Autodesk Inventor part; units mm, degrees
(part 3 of 4)
  line L1059 (-6.67, 65.7894) -> (-6.9506, 66.0778) construction
  line L1060 (-6.9506, 66.0778) -> (-7.1688, 66.0778) construction
  spline S276 degree 2 poles (-8.1665, 63.3342) (-8.1665, 63.2173) (-8.2366, 63.1472) knots 0 0 0 1 1 1
  line L1061 (-8.1665, 63.3342) -> (-8.1665, 63.2173) construction
  line L1062 (-8.1665, 63.2173) -> (-8.2366, 63.1472) construction
  spline S277 degree 2 poles (-8.2366, 63.1472) (-8.3068, 63.0848) (-8.4159, 63.0848) knots 0 0 0 1 1 1
  line L1063 (-8.2366, 63.1472) -> (-8.3068, 63.0848) construction
  line L1064 (-8.3068, 63.0848) -> (-8.4159, 63.0848) construction
  spline S278 degree 2 poles (-8.4159, 63.0848) (-8.5172, 63.0848) (-8.6653, 63.2095) (-8.6653, 63.3342) knots 0 0 0 1 2 2 2
  line L1065 (-8.4159, 63.0848) -> (-8.5172, 63.0848) construction
  line L1066 (-8.5172, 63.0848) -> (-8.6653, 63.2095) construction
  line L1067 (-8.6653, 63.2095) -> (-8.6653, 63.3342) construction
  line L1068 (-8.6653, 63.3342) -> (-8.6653, 66.3272)
  spline S279 degree 2 poles (-8.6653, 66.3272) (-8.6653, 66.5766) (-8.4159, 66.5766) knots 0 0 0 1 1 1
  line L1069 (-8.6653, 66.3272) -> (-8.6653, 66.5766) construction
  line L1070 (-8.6653, 66.5766) -> (-8.4159, 66.5766) construction
  line L1071 (-8.4159, 66.5766) -> (-7.1688, 66.5766)
  spline S280 degree 2 poles (-7.1688, 66.5766) (-6.7713, 66.5766) (-6.1712, 66.0038) (-6.1712, 65.579) knots 0 0 0 1 2 2 2
  line L1072 (-7.1688, 66.5766) -> (-6.7713, 66.5766) construction
  line L1073 (-6.7713, 66.5766) -> (-6.1712, 66.0038) construction
  line L1074 (-6.1712, 66.0038) -> (-6.1712, 65.579) construction
  line L1075 (-6.1712, 65.579) -> (-6.1712, 63.3342)
  spline S281 degree 2 poles (-6.1712, 63.3342) (-6.1712, 63.2173) (-6.2413, 63.1472) knots 0 0 0 1 1 1
  line L1076 (-6.1712, 63.3342) -> (-6.1712, 63.2173) construction
  line L1077 (-6.1712, 63.2173) -> (-6.2413, 63.1472) construction
  spline S282 degree 2 poles (2.309, 64.0825) (2.309, 63.872) (2.4532, 63.7278) knots 0 0 0 1 1 1
  line L1078 (2.309, 64.0825) -> (2.309, 63.872) construction
  line L1079 (2.309, 63.872) -> (2.4532, 63.7278) construction
  spline S283 degree 2 poles (2.4532, 63.7278) (2.5272, 63.6616) (2.6129, 63.6187) knots 0 0 0 1 1 1
  line L1080 (2.4532, 63.7278) -> (2.5272, 63.6616) construction
  line L1081 (2.5272, 63.6616) -> (2.6129, 63.6187) construction
  spline S284 degree 2 poles (2.6129, 63.6187) (2.7182, 63.5836) (2.8078, 63.5836) knots 0 0 0 1 1 1
  line L1082 (2.6129, 63.6187) -> (2.7182, 63.5836) construction
  line L1083 (2.7182, 63.5836) -> (2.8078, 63.5836) construction
  line L1084 (2.8078, 63.5836) -> (4.0549, 63.5836)
  spline S285 degree 2 poles (4.0549, 63.5836) (4.1601, 63.5836) (4.3043, 63.4317) (4.3043, 63.3342) knots 0 0 0 1 2 2 2
  line L1085 (4.0549, 63.5836) -> (4.1601, 63.5836) construction
  line L1086 (4.1601, 63.5836) -> (4.3043, 63.4317) construction
  line L1087 (4.3043, 63.4317) -> (4.3043, 63.3342) construction
  spline S286 degree 2 poles (4.3043, 63.3342) (4.3043, 63.2485) (4.1796, 63.0848) (4.0549, 63.0848) knots 0 0 0 1 2 2 2
  line L1088 (4.3043, 63.3342) -> (4.3043, 63.2485) construction
  line L1089 (4.3043, 63.2485) -> (4.1796, 63.0848) construction
  line L1090 (4.1796, 63.0848) -> (4.0549, 63.0848) construction
  line L1091 (4.0549, 63.0848) -> (2.8078, 63.0848)
  spline S287 degree 2 poles (2.8078, 63.0848) (2.4025, 63.0848) (1.8101, 63.6655) (1.8101, 64.0825) knots 0 0 0 1 2 2 2
  line L1092 (2.8078, 63.0848) -> (2.4025, 63.0848) construction
  line L1093 (2.4025, 63.0848) -> (1.8101, 63.6655) construction
  line L1094 (1.8101, 63.6655) -> (1.8101, 64.0825) construction
  line L1095 (1.8101, 64.0825) -> (1.8101, 65.579)
  spline S288 degree 2 poles (1.8101, 65.579) (1.8101, 65.9804) (2.3869, 66.5766) (2.8078, 66.5766) knots 0 0 0 1 2 2 2
  line L1096 (1.8101, 65.579) -> (1.8101, 65.9804) construction
  line L1097 (1.8101, 65.9804) -> (2.3869, 66.5766) construction
  line L1098 (2.3869, 66.5766) -> (2.8078, 66.5766) construction
  line L1099 (2.8078, 66.5766) -> (3.3066, 66.5766)
  spline S289 degree 2 poles (3.3066, 66.5766) (3.7119, 66.5766) (4.3043, 65.996) (4.3043, 65.579) knots 0 0 0 1 2 2 2
  line L1100 (3.3066, 66.5766) -> (3.7119, 66.5766) construction
  line L1101 (3.7119, 66.5766) -> (4.3043, 65.996) construction
  line L1102 (4.3043, 65.996) -> (4.3043, 65.579) construction
  line L1103 (4.3043, 65.579) -> (4.3043, 64.8307)
  spline S290 degree 2 poles (4.3043, 64.8307) (4.3043, 64.5813) (4.0549, 64.5813) knots 0 0 0 1 1 1
  line L1104 (4.3043, 64.8307) -> (4.3043, 64.5813) construction
  line L1105 (4.3043, 64.5813) -> (4.0549, 64.5813) construction
  spline S291 degree 2 poles (5.8008, 63.3342) (5.8008, 63.2173) (5.7306, 63.1472) knots 0 0 0 1 1 1
  line L1106 (5.8008, 63.3342) -> (5.8008, 63.2173) construction
  line L1107 (5.8008, 63.2173) -> (5.7306, 63.1472) construction
  spline S292 degree 2 poles (5.7306, 63.1472) (5.6605, 63.0848) (5.5514, 63.0848) knots 0 0 0 1 1 1
  line L1108 (5.7306, 63.1472) -> (5.6605, 63.0848) construction
  line L1109 (5.6605, 63.0848) -> (5.5514, 63.0848) construction
  spline S293 degree 2 poles (5.5514, 63.0848) (5.45, 63.0848) (5.302, 63.2095) (5.302, 63.3342) knots 0 0 0 1 2 2 2
  line L1110 (5.5514, 63.0848) -> (5.45, 63.0848) construction
  line L1111 (5.45, 63.0848) -> (5.302, 63.2095) construction
  line L1112 (5.302, 63.2095) -> (5.302, 63.3342) construction
  line L1113 (5.302, 63.3342) -> (5.302, 66.3272)
  spline S294 degree 2 poles (5.302, 66.3272) (5.302, 66.5766) (5.5514, 66.5766) knots 0 0 0 1 1 1
  line L1114 (5.302, 66.3272) -> (5.302, 66.5766) construction
  line L1115 (5.302, 66.5766) -> (5.5514, 66.5766) construction
  line L1116 (5.5514, 66.5766) -> (7.7961, 66.5766)
  spline S295 degree 2 poles (7.7961, 66.5766) (8.2014, 66.5766) (8.7938, 65.996) (8.7938, 65.579) knots 0 0 0 1 2 2 2
  line L1117 (7.7961, 66.5766) -> (8.2014, 66.5766) construction
  line L1118 (8.2014, 66.5766) -> (8.7938, 65.996) construction
  line L1119 (8.7938, 65.996) -> (8.7938, 65.579) construction
  line L1120 (8.7938, 65.579) -> (8.7938, 63.3342)
  spline S296 degree 2 poles (8.7938, 63.3342) (8.7938, 63.2173) (8.7236, 63.1472) knots 0 0 0 1 1 1
  line L1121 (8.7938, 63.3342) -> (8.7938, 63.2173) construction
  line L1122 (8.7938, 63.2173) -> (8.7236, 63.1472) construction
  spline S297 degree 2 poles (8.7236, 63.1472) (8.6535, 63.0848) (8.5444, 63.0848) knots 0 0 0 1 1 1
  line L1123 (8.7236, 63.1472) -> (8.6535, 63.0848) construction
  line L1124 (8.6535, 63.0848) -> (8.5444, 63.0848) construction
  spline S298 degree 2 poles (8.5444, 63.0848) (8.443, 63.0848) (8.2949, 63.2095) (8.2949, 63.3342) knots 0 0 0 1 2 2 2
  line L1125 (8.5444, 63.0848) -> (8.443, 63.0848) construction
  line L1126 (8.443, 63.0848) -> (8.2949, 63.2095) construction
  line L1127 (8.2949, 63.2095) -> (8.2949, 63.3342) construction
  line L1128 (8.2949, 63.3342) -> (8.2949, 65.579)
  spline S299 degree 2 poles (8.2949, 65.579) (8.2949, 65.7894) (8.0143, 66.0778) (7.7961, 66.0778) knots 0 0 0 1 2 2 2
  line L1129 (8.2949, 65.579) -> (8.2949, 65.7894) construction
  line L1130 (8.2949, 65.7894) -> (8.0143, 66.0778) construction
  line L1131 (8.0143, 66.0778) -> (7.7961, 66.0778) construction
  spline S300 degree 2 poles (7.2973, 63.3342) (7.2973, 63.2173) (7.2271, 63.1472) knots 0 0 0 1 1 1
  line L1132 (7.2973, 63.3342) -> (7.2973, 63.2173) construction
  line L1133 (7.2973, 63.2173) -> (7.2271, 63.1472) construction
  spline S301 degree 2 poles (7.2271, 63.1472) (7.157, 63.0848) (7.0479, 63.0848) knots 0 0 0 1 1 1
  line L1134 (7.2271, 63.1472) -> (7.157, 63.0848) construction
  line L1135 (7.157, 63.0848) -> (7.0479, 63.0848) construction
  spline S302 degree 2 poles (7.0479, 63.0848) (6.9465, 63.0848) (6.7984, 63.2095) (6.7984, 63.3342) knots 0 0 0 1 2 2 2
  line L1136 (7.0479, 63.0848) -> (6.9465, 63.0848) construction
  line L1137 (6.9465, 63.0848) -> (6.7984, 63.2095) construction
  line L1138 (6.7984, 63.2095) -> (6.7984, 63.3342) construction
  spline S303 degree 2 poles (1.346, 31.5891) (1.346, 31.4722) (1.1862, 31.3397) (1.0966, 31.3397) knots -2 -2 -2 -1 0 0 0
  line L1139 (1.346, 31.5891) -> (1.346, 31.4722) construction
  line L1140 (1.346, 31.4722) -> (1.1862, 31.3397) construction
  line L1141 (1.1862, 31.3397) -> (1.0966, 31.3397) construction
  spline S304 degree 2 poles (1.0966, 31.3397) (0.9875, 31.3397) (0.9173, 31.4021) knots -1 -1 -1 0 0 0
  line L1142 (1.0966, 31.3397) -> (0.9875, 31.3397) construction
  line L1143 (0.9875, 31.3397) -> (0.9173, 31.4021) construction
  spline S305 degree 2 poles (0.9173, 31.4021) (0.8472, 31.4722) (0.8472, 31.5891) knots -1 -1 -1 0 0 0
  line L1144 (0.9173, 31.4021) -> (0.8472, 31.4722) construction
  line L1145 (0.8472, 31.4722) -> (0.8472, 31.5891) construction
  spline S306 degree 2 poles (0.0521, 32.692) (-0.0531, 32.5595) (-0.1505, 32.5595) knots -1 -1 -1 0 0 0
  line L1146 (0.0521, 32.692) -> (-0.0531, 32.5595) construction
  line L1147 (-0.0531, 32.5595) -> (-0.1505, 32.5595) construction
  spline S307 degree 2 poles (-0.1505, 32.5595) (-0.2557, 32.5595) (-0.3532, 32.692) knots -1 -1 -1 0 0 0
  line L1148 (-0.1505, 32.5595) -> (-0.2557, 32.5595) construction
  line L1149 (-0.2557, 32.5595) -> (-0.3532, 32.692) construction
  spline S308 degree 2 poles (-1.1482, 31.5891) (-1.1482, 31.4722) (-1.3079, 31.3397) (-1.3976, 31.3397) knots -2 -2 -2 -1 0 0 0
  line L1150 (-1.1482, 31.5891) -> (-1.1482, 31.4722) construction
  line L1151 (-1.1482, 31.4722) -> (-1.3079, 31.3397) construction
  line L1152 (-1.3079, 31.3397) -> (-1.3976, 31.3397) construction
  spline S309 degree 2 poles (-1.3976, 31.3397) (-1.5067, 31.3397) (-1.5768, 31.4021) knots -1 -1 -1 0 0 0
  line L1153 (-1.3976, 31.3397) -> (-1.5067, 31.3397) construction
  line L1154 (-1.5067, 31.3397) -> (-1.5768, 31.4021) construction
  spline S310 degree 2 poles (-1.5768, 31.4021) (-1.647, 31.4722) (-1.647, 31.5891) knots -1 -1 -1 0 0 0
  line L1155 (-1.5768, 31.4021) -> (-1.647, 31.4722) construction
  line L1156 (-1.647, 31.4722) -> (-1.647, 31.5891) construction
  line L1157 (-1.647, 31.5891) -> (-1.647, 34.5821)
  spline S311 degree 2 poles (-1.647, 34.5821) (-1.647, 34.7146) (-1.5846, 34.7926) knots -1 -1 -1 0 0 0
  line L1158 (-1.647, 34.5821) -> (-1.647, 34.7146) construction
  line L1159 (-1.647, 34.7146) -> (-1.5846, 34.7926) construction
  spline S312 degree 2 poles (-1.5846, 34.7926) (-1.5106, 34.8705) (-1.4249, 34.8705) knots -1 -1 -1 0 0 0
  line L1160 (-1.5846, 34.7926) -> (-1.5106, 34.8705) construction
  line L1161 (-1.5106, 34.8705) -> (-1.4249, 34.8705) construction
  spline S313 degree 2 poles (-1.4249, 34.8705) (-1.2924, 34.8705) (-1.1949, 34.7263) knots -1 -1 -1 0 0 0
  line L1162 (-1.4249, 34.8705) -> (-1.2924, 34.8705) construction
  line L1163 (-1.2924, 34.8705) -> (-1.1949, 34.7263) construction
  spline S314 degree 2 poles (0.8939, 34.7263) (1.0147, 34.8705) (1.1239, 34.8705) knots -1 -1 -1 0 0 0
  line L1164 (0.8939, 34.7263) -> (1.0147, 34.8705) construction
  line L1165 (1.0147, 34.8705) -> (1.1239, 34.8705) construction
  spline S315 degree 2 poles (1.1239, 34.8705) (1.2174, 34.8705) (1.346, 34.7224) (1.346, 34.5821) knots -2 -2 -2 -1 0 0 0
  line L1166 (1.1239, 34.8705) -> (1.2174, 34.8705) construction
  line L1167 (1.2174, 34.8705) -> (1.346, 34.7224) construction
  line L1168 (1.346, 34.7224) -> (1.346, 34.5821) construction
  line L1169 (1.346, 34.5821) -> (1.346, 31.5891)
  line L1170 (10.8238, 31.3397) -> (10.3249, 31.3397)
  spline S316 degree 2 poles (10.3249, 31.3397) (9.9235, 31.3397) (9.3273, 31.9165) (9.3273, 32.3374) knots 0 0 0 1 2 2 2
  line L1171 (10.3249, 31.3397) -> (9.9235, 31.3397) construction
  line L1172 (9.9235, 31.3397) -> (9.3273, 31.9165) construction
  line L1173 (9.3273, 31.9165) -> (9.3273, 32.3374) construction
  line L1174 (9.3273, 32.3374) -> (9.3273, 33.8339)
  spline S317 degree 2 poles (9.3273, 33.8339) (9.3273, 34.247) (9.9119, 34.8315) (10.3249, 34.8315) knots 0 0 0 1 2 2 2
  line L1175 (9.3273, 33.8339) -> (9.3273, 34.247) construction
  line L1176 (9.3273, 34.247) -> (9.9119, 34.8315) construction
  line L1177 (9.9119, 34.8315) -> (10.3249, 34.8315) construction
  line L1178 (10.3249, 34.8315) -> (11.572, 34.8315)
  spline S318 degree 2 poles (11.572, 34.8315) (11.8214, 34.8315) (11.8214, 34.5821) knots 0 0 0 1 1 1
  line L1179 (11.572, 34.8315) -> (11.8214, 34.8315) construction
  line L1180 (11.8214, 34.8315) -> (11.8214, 34.5821) construction
  line L1181 (11.8214, 34.5821) -> (11.8214, 32.3452)
  spline S319 degree 2 poles (11.8214, 32.3452) (11.8214, 32.1932) (11.9189, 32.0373) knots 0 0 0 1 1 1
  line L1182 (11.8214, 32.3452) -> (11.8214, 32.1932) construction
  line L1183 (11.8214, 32.1932) -> (11.9189, 32.0373) construction
  spline S320 degree 2 poles (11.9189, 32.0373) (12.0046, 31.897) (12.1683, 31.8191) knots 0 0 0 1 1 1
  line L1184 (11.9189, 32.0373) -> (12.0046, 31.897) construction
  line L1185 (12.0046, 31.897) -> (12.1683, 31.8191) construction
  spline S321 degree 2 poles (12.1683, 31.8191) (12.3242, 31.7567) (12.3242, 31.5969) knots 0 0 0 1 1 1
  line L1186 (12.1683, 31.8191) -> (12.3242, 31.7567) construction
  line L1187 (12.3242, 31.7567) -> (12.3242, 31.5969) construction
  spline S322 degree 2 poles (12.3242, 31.5969) (12.3242, 31.4839) (12.2501, 31.4138) knots 0 0 0 1 1 1
  line L1188 (12.3242, 31.5969) -> (12.3242, 31.4839) construction
  line L1189 (12.3242, 31.4839) -> (12.2501, 31.4138) construction
  spline S323 degree 2 poles (12.2501, 31.4138) (12.1878, 31.3397) (12.0748, 31.3397) knots 0 0 0 1 1 1
  line L1190 (12.2501, 31.4138) -> (12.1878, 31.3397) construction
  line L1191 (12.1878, 31.3397) -> (12.0748, 31.3397) construction
  spline S324 degree 2 poles (12.0748, 31.3397) (12.0202, 31.3397) (11.9695, 31.3631) knots 0 0 0 1 1 1
  line L1192 (12.0748, 31.3397) -> (12.0202, 31.3397) construction
  line L1193 (12.0202, 31.3397) -> (11.9695, 31.3631) construction
  spline S325 degree 2 poles (11.9695, 31.3631) (11.724, 31.4605) (11.5681, 31.6671) knots 0 0 0 1 1 1
  line L1194 (11.9695, 31.3631) -> (11.724, 31.4605) construction
  line L1195 (11.724, 31.4605) -> (11.5681, 31.6671) construction
  spline S326 degree 2 poles (11.5681, 31.6671) (11.4473, 31.5268) (11.0303, 31.3397) (10.8238, 31.3397) knots 0 0 0 1 2 2 2
  line L1196 (11.5681, 31.6671) -> (11.4473, 31.5268) construction
  line L1197 (11.4473, 31.5268) -> (11.0303, 31.3397) construction
  line L1198 (11.0303, 31.3397) -> (10.8238, 31.3397) construction
  spline S327 degree 2 poles (-4.4607, 27.316) (-4.5309, 27.2537) (-4.64, 27.2537) knots 0 0 0 1 1 1
  line L1199 (-4.4607, 27.316) -> (-4.5309, 27.2537) construction
  line L1200 (-4.5309, 27.2537) -> (-4.64, 27.2537) construction
  spline S328 degree 2 poles (-4.64, 27.2537) (-4.7413, 27.2537) (-4.8894, 27.3784) (-4.8894, 27.5031) knots 0 0 0 1 2 2 2
  line L1201 (-4.64, 27.2537) -> (-4.7413, 27.2537) construction
  line L1202 (-4.7413, 27.2537) -> (-4.8894, 27.3784) construction
  line L1203 (-4.8894, 27.3784) -> (-4.8894, 27.5031) construction
  line L1204 (-4.8894, 27.5031) -> (-4.8894, 29.7478)
  spline S329 degree 2 poles (-4.8894, 29.7478) (-4.8894, 29.9583) (-5.17, 30.2467) (-5.3882, 30.2467) knots 0 0 0 1 2 2 2
  line L1205 (-4.8894, 29.7478) -> (-4.8894, 29.9583) construction
  line L1206 (-4.8894, 29.9583) -> (-5.17, 30.2467) construction
  line L1207 (-5.17, 30.2467) -> (-5.3882, 30.2467) construction
  spline S330 degree 2 poles (-6.3859, 27.5031) (-6.3859, 27.3862) (-6.456, 27.316) knots 0 0 0 1 1 1
  line L1208 (-6.3859, 27.5031) -> (-6.3859, 27.3862) construction
  line L1209 (-6.3859, 27.3862) -> (-6.456, 27.316) construction
  spline S331 degree 2 poles (-6.456, 27.316) (-6.5262, 27.2537) (-6.6353, 27.2537) knots 0 0 0 1 1 1
  line L1210 (-6.456, 27.316) -> (-6.5262, 27.2537) construction
  line L1211 (-6.5262, 27.2537) -> (-6.6353, 27.2537) construction
  spline S332 degree 2 poles (-6.6353, 27.2537) (-6.7366, 27.2537) (-6.8847, 27.3784) (-6.8847, 27.5031) knots 0 0 0 1 2 2 2
  line L1212 (-6.6353, 27.2537) -> (-6.7366, 27.2537) construction
  line L1213 (-6.7366, 27.2537) -> (-6.8847, 27.3784) construction
  line L1214 (-6.8847, 27.3784) -> (-6.8847, 27.5031) construction
  line L1215 (-6.8847, 27.5031) -> (-6.8847, 30.4961)
  spline S333 degree 2 poles (-6.8847, 30.4961) (-6.8847, 30.7455) (-6.6353, 30.7455) knots 0 0 0 1 1 1
  line L1216 (-6.8847, 30.4961) -> (-6.8847, 30.7455) construction
  line L1217 (-6.8847, 30.7455) -> (-6.6353, 30.7455) construction
  line L1218 (-6.6353, 30.7455) -> (-5.3882, 30.7455)
  spline S334 degree 2 poles (-5.3882, 30.7455) (-4.9907, 30.7455) (-4.3906, 30.1726) (-4.3906, 29.7478) knots 0 0 0 1 2 2 2
  line L1219 (-5.3882, 30.7455) -> (-4.9907, 30.7455) construction
  line L1220 (-4.9907, 30.7455) -> (-4.3906, 30.1726) construction
  line L1221 (-4.3906, 30.1726) -> (-4.3906, 29.7478) construction
  line L1222 (-4.3906, 29.7478) -> (-4.3906, 27.5031)
  spline S335 degree 2 poles (-4.3906, 27.5031) (-4.3906, 27.3862) (-4.4607, 27.316) knots 0 0 0 1 1 1
  line L1223 (-4.3906, 27.5031) -> (-4.3906, 27.3862) construction
  line L1224 (-4.3906, 27.3862) -> (-4.4607, 27.316) construction
  spline S336 degree 2 poles (1.0966, 27.2537) (0.6952, 27.2537) (0.0989, 27.8305) (0.0989, 28.2513) knots 0 0 0 1 2 2 2
  line L1225 (1.0966, 27.2537) -> (0.6952, 27.2537) construction
  line L1226 (0.6952, 27.2537) -> (0.0989, 27.8305) construction
  line L1227 (0.0989, 27.8305) -> (0.0989, 28.2513) construction
  line L1228 (0.0989, 28.2513) -> (0.0989, 29.7478)
  spline S337 degree 2 poles (0.0989, 29.7478) (0.0989, 30.1609) (0.6835, 30.7455) (1.0966, 30.7455) knots 0 0 0 1 2 2 2
  line L1229 (0.0989, 29.7478) -> (0.0989, 30.1609) construction
  line L1230 (0.0989, 30.1609) -> (0.6835, 30.7455) construction
  line L1231 (0.6835, 30.7455) -> (1.0966, 30.7455) construction
  line L1232 (1.0966, 30.7455) -> (1.8448, 30.7455)
  spline S338 degree 2 poles (1.8448, 30.7455) (1.9461, 30.7455) (2.0942, 30.5935) (2.0942, 30.4961) knots 0 0 0 1 2 2 2
  line L1233 (1.8448, 30.7455) -> (1.9461, 30.7455) construction
  line L1234 (1.9461, 30.7455) -> (2.0942, 30.5935) construction
  line L1235 (2.0942, 30.5935) -> (2.0942, 30.4961) construction
  spline S339 degree 2 poles (2.0942, 30.4961) (2.0942, 30.4103) (1.9695, 30.2467) (1.8448, 30.2467) knots 0 0 0 1 2 2 2
  line L1236 (2.0942, 30.4961) -> (2.0942, 30.4103) construction
  line L1237 (2.0942, 30.4103) -> (1.9695, 30.2467) construction
  line L1238 (1.9695, 30.2467) -> (1.8448, 30.2467) construction
  line L1239 (1.8448, 30.2467) -> (1.0966, 30.2467)
  spline S340 degree 2 poles (1.0966, 30.2467) (0.8861, 30.2467) (0.7419, 30.1025) knots 0 0 0 1 1 1
  line L1240 (1.0966, 30.2467) -> (0.8861, 30.2467) construction
  line L1241 (0.8861, 30.2467) -> (0.7419, 30.1025) construction
  spline S341 degree 2 poles (0.7419, 30.1025) (0.6679, 30.0323) (0.5977, 29.8531) (0.5977, 29.7478) knots 0 0 0 1 2 2 2
  line L1242 (0.7419, 30.1025) -> (0.6679, 30.0323) construction
  line L1243 (0.6679, 30.0323) -> (0.5977, 29.8531) construction
  line L1244 (0.5977, 29.8531) -> (0.5977, 29.7478) construction
  line L1245 (0.5977, 29.7478) -> (0.5977, 28.2513)
  spline S342 degree 2 poles (0.5977, 28.2513) (0.5977, 28.0409) (0.7419, 27.8967) knots 0 0 0 1 1 1
  line L1246 (0.5977, 28.2513) -> (0.5977, 28.0409) construction
  line L1247 (0.5977, 28.0409) -> (0.7419, 27.8967) construction
  spline S343 degree 2 poles (0.7419, 27.8967) (0.816, 27.8305) (0.9017, 27.7876) knots 0 0 0 1 1 1
  line L1248 (0.7419, 27.8967) -> (0.816, 27.8305) construction
  line L1249 (0.816, 27.8305) -> (0.9017, 27.7876) construction
  spline S344 degree 2 poles (0.9017, 27.7876) (1.0069, 27.7525) (1.0966, 27.7525) knots 0 0 0 1 1 1
  line L1250 (0.9017, 27.7876) -> (1.0069, 27.7525) construction
  line L1251 (1.0069, 27.7525) -> (1.0966, 27.7525) construction
  line L1252 (1.0966, 27.7525) -> (1.8448, 27.7525)
  spline S345 degree 2 poles (1.8448, 27.7525) (1.9461, 27.7525) (2.0942, 27.6005) (2.0942, 27.5031) knots 0 0 0 1 2 2 2
  line L1253 (1.8448, 27.7525) -> (1.9461, 27.7525) construction
  line L1254 (1.9461, 27.7525) -> (2.0942, 27.6005) construction
  line L1255 (2.0942, 27.6005) -> (2.0942, 27.5031) construction
  spline S346 degree 2 poles (2.0942, 27.5031) (2.0942, 27.4174) (1.9695, 27.2537) (1.8448, 27.2537) knots 0 0 0 1 2 2 2
  line L1256 (2.0942, 27.5031) -> (2.0942, 27.4174) construction
  line L1257 (2.0942, 27.4174) -> (1.9695, 27.2537) construction
  line L1258 (1.9695, 27.2537) -> (1.8448, 27.2537) construction
  line L1259 (1.8448, 27.2537) -> (1.0966, 27.2537)
  line L1260 (8.0802, 27.2537) -> (7.5814, 27.2537)
  spline S347 degree 2 poles (7.5814, 27.2537) (7.18, 27.2537) (6.5837, 27.8305) (6.5837, 28.2513) knots 0 0 0 1 2 2 2
  line L1261 (7.5814, 27.2537) -> (7.18, 27.2537) construction
  line L1262 (7.18, 27.2537) -> (6.5837, 27.8305) construction
  line L1263 (6.5837, 27.8305) -> (6.5837, 28.2513) construction
  line L1264 (6.5837, 28.2513) -> (6.5837, 29.7478)
  spline S348 degree 2 poles (6.5837, 29.7478) (6.5837, 30.1609) (7.1683, 30.7455) (7.5814, 30.7455) knots 0 0 0 1 2 2 2
  line L1265 (6.5837, 29.7478) -> (6.5837, 30.1609) construction
  line L1266 (6.5837, 30.1609) -> (7.1683, 30.7455) construction
  line L1267 (7.1683, 30.7455) -> (7.5814, 30.7455) construction
  line L1268 (7.5814, 30.7455) -> (8.8285, 30.7455)
  spline S349 degree 2 poles (8.8285, 30.7455) (9.0779, 30.7455) (9.0779, 30.4961) knots 0 0 0 1 1 1
  line L1269 (8.8285, 30.7455) -> (9.0779, 30.7455) construction
  line L1270 (9.0779, 30.7455) -> (9.0779, 30.4961) construction
  line L1271 (9.0779, 30.4961) -> (9.0779, 28.2591)
  spline S350 degree 2 poles (9.0779, 28.2591) (9.0779, 28.1072) (9.1753, 27.9513) knots 0 0 0 1 1 1
  line L1272 (9.0779, 28.2591) -> (9.0779, 28.1072) construction
  line L1273 (9.0779, 28.1072) -> (9.1753, 27.9513) construction
  spline S351 degree 2 poles (9.1753, 27.9513) (9.261, 27.811) (9.4247, 27.733) knots 0 0 0 1 1 1
  line L1274 (9.1753, 27.9513) -> (9.261, 27.811) construction
  line L1275 (9.261, 27.811) -> (9.4247, 27.733) construction
  spline S352 degree 2 poles (9.4247, 27.733) (9.5806, 27.6707) (9.5806, 27.5109) knots 0 0 0 1 1 1
  line L1276 (9.4247, 27.733) -> (9.5806, 27.6707) construction
  line L1277 (9.5806, 27.6707) -> (9.5806, 27.5109) construction
  spline S353 degree 2 poles (9.5806, 27.5109) (9.5806, 27.3979) (9.5066, 27.3277) knots 0 0 0 1 1 1
  line L1278 (9.5806, 27.5109) -> (9.5806, 27.3979) construction
  line L1279 (9.5806, 27.3979) -> (9.5066, 27.3277) construction
  spline S354 degree 2 poles (9.5066, 27.3277) (9.4442, 27.2537) (9.3312, 27.2537) knots 0 0 0 1 1 1
  line L1280 (9.5066, 27.3277) -> (9.4442, 27.2537) construction
  line L1281 (9.4442, 27.2537) -> (9.3312, 27.2537) construction
  spline S355 degree 2 poles (9.3312, 27.2537) (9.2766, 27.2537) (9.226, 27.2771) knots 0 0 0 1 1 1
  line L1282 (9.3312, 27.2537) -> (9.2766, 27.2537) construction
  line L1283 (9.2766, 27.2537) -> (9.226, 27.2771) construction
  spline S356 degree 2 poles (9.226, 27.2771) (8.9804, 27.3745) (8.8246, 27.581) knots 0 0 0 1 1 1
  line L1284 (9.226, 27.2771) -> (8.9804, 27.3745) construction
  line L1285 (8.9804, 27.3745) -> (8.8246, 27.581) construction
  spline S357 degree 2 poles (8.8246, 27.581) (8.7037, 27.4407) (8.2868, 27.2537) (8.0802, 27.2537) knots 0 0 0 1 2 2 2
  line L1286 (8.8246, 27.581) -> (8.7037, 27.4407) construction
  line L1287 (8.7037, 27.4407) -> (8.2868, 27.2537) construction
  line L1288 (8.2868, 27.2537) -> (8.0802, 27.2537) construction
  line L1289 (-34.888, -102.8274) -> (-35.1278, -102.8274)
  spline S358 degree 2 poles (-35.1278, -102.8274) (-35.4875, -102.8274) (-36.0037, -102.3145) (-36.0037, -101.9514) knots 0 0 0 1 2 2 2
  line L1290 (-35.1278, -102.8274) -> (-35.4875, -102.8274) construction
  line L1291 (-35.4875, -102.8274) -> (-36.0037, -102.3145) construction
  line L1292 (-36.0037, -102.3145) -> (-36.0037, -101.9514) construction
  line L1293 (-36.0037, -101.9514) -> (-36.0037, -100.9123)
  spline S359 degree 2 poles (-36.0037, -100.9123) (-36.0037, -100.5493) (-35.4875, -100.0364) (-35.1278, -100.0364) knots 0 0 0 1 2 2 2
  line L1294 (-36.0037, -100.9123) -> (-36.0037, -100.5493) construction
  line L1295 (-36.0037, -100.5493) -> (-35.4875, -100.0364) construction
  line L1296 (-35.4875, -100.0364) -> (-35.1278, -100.0364) construction
  line L1297 (-35.1278, -100.0364) -> (-34.888, -100.0364)
  spline S360 degree 2 poles (-34.888, -100.0364) (-34.525, -100.0364) (-34.012, -100.5493) (-34.012, -100.9123) knots 0 0 0 1 2 2 2
  line L1298 (-34.888, -100.0364) -> (-34.525, -100.0364) construction
  line L1299 (-34.525, -100.0364) -> (-34.012, -100.5493) construction
  line L1300 (-34.012, -100.5493) -> (-34.012, -100.9123) construction
  line L1301 (-34.012, -100.9123) -> (-34.012, -101.9514)
  spline S361 degree 2 poles (-34.012, -101.9514) (-34.012, -102.3178) (-34.525, -102.8274) (-34.888, -102.8274) knots 0 0 0 1 2 2 2
  line L1302 (-34.012, -101.9514) -> (-34.012, -102.3178) construction
  line L1303 (-34.012, -102.3178) -> (-34.525, -102.8274) construction
  line L1304 (-34.525, -102.8274) -> (-34.888, -102.8274) construction
  spline S362 degree 2 poles (-32.813, -102.6276) (-32.813, -102.8274) (-33.0129, -102.8274) knots 0 0 0 1 1 1
  line L1305 (-32.813, -102.6276) -> (-32.813, -102.8274) construction
  line L1306 (-32.813, -102.8274) -> (-33.0129, -102.8274) construction
  spline S363 degree 2 poles (-33.0129, -102.8274) (-33.2127, -102.8274) (-33.2127, -102.6276) knots 0 0 0 1 1 1
  line L1307 (-33.0129, -102.8274) -> (-33.2127, -102.8274) construction
  line L1308 (-33.2127, -102.8274) -> (-33.2127, -102.6276) construction
  line L1309 (-33.2127, -102.6276) -> (-33.2127, -100.2362)
  spline S364 degree 2 poles (-33.2127, -100.2362) (-33.2127, -100.0364) (-33.0129, -100.0364) knots 0 0 0 1 1 1
  line L1310 (-33.2127, -100.2362) -> (-33.2127, -100.0364) construction
  line L1311 (-33.2127, -100.0364) -> (-33.0129, -100.0364) construction
  line L1312 (-33.0129, -100.0364) -> (-31.2177, -100.0364)
  spline S365 degree 2 poles (-31.2177, -100.0364) (-30.888, -100.0364) (-30.4217, -100.5027) (-30.4217, -100.8324) knots 0 0 0 1 2 2 2
  line L1313 (-31.2177, -100.0364) -> (-30.888, -100.0364) construction
  line L1314 (-30.888, -100.0364) -> (-30.4217, -100.5027) construction
  line L1315 (-30.4217, -100.5027) -> (-30.4217, -100.8324) construction
  line L1316 (-30.4217, -100.8324) -> (-30.4217, -102.6276)
  spline S366 degree 2 poles (-30.4217, -102.6276) (-30.4217, -102.8274) (-30.6215, -102.8274) knots 0 0 0 1 1 1
  line L1317 (-30.4217, -102.6276) -> (-30.4217, -102.8274) construction
  line L1318 (-30.4217, -102.8274) -> (-30.6215, -102.8274) construction
  spline S367 degree 2 poles (-30.6215, -102.8274) (-30.8214, -102.8274) (-30.8214, -102.6276) knots 0 0 0 1 1 1
  line L1319 (-30.6215, -102.8274) -> (-30.8214, -102.8274) construction
  line L1320 (-30.8214, -102.8274) -> (-30.8214, -102.6276) construction
  line L1321 (-30.8214, -102.6276) -> (-30.8214, -100.8357)
  spline S368 degree 2 poles (-30.8214, -100.8357) (-30.8214, -100.6725) (-31.0545, -100.436) (-31.2177, -100.436) knots 0 0 0 1 2 2 2
  line L1322 (-30.8214, -100.8357) -> (-30.8214, -100.6725) construction
  line L1323 (-30.8214, -100.6725) -> (-31.0545, -100.436) construction
  line L1324 (-31.0545, -100.436) -> (-31.2177, -100.436) construction
  spline S369 degree 2 poles (-31.6174, -102.6276) (-31.6174, -102.8274) (-31.8172, -102.8274) knots 0 0 0 1 1 1
  line L1325 (-31.6174, -102.6276) -> (-31.6174, -102.8274) construction
  line L1326 (-31.6174, -102.8274) -> (-31.8172, -102.8274) construction
  spline S370 degree 2 poles (-31.8172, -102.8274) (-32.017, -102.8274) (-32.017, -102.6276) knots 0 0 0 1 1 1
  line L1327 (-31.8172, -102.8274) -> (-32.017, -102.8274) construction
  line L1328 (-32.017, -102.8274) -> (-32.017, -102.6276) construction
  spline S371 degree 2 poles (-24.6399, -102.8274) (-24.8397, -102.8274) (-24.8397, -102.6276) knots 0 0 0 1 1 1
  line L1329 (-24.6399, -102.8274) -> (-24.8397, -102.8274) construction
  line L1330 (-24.8397, -102.8274) -> (-24.8397, -102.6276) construction
  line L1331 (-24.8397, -102.6276) -> (-24.8397, -100.2362)
  spline S372 degree 2 poles (-24.8397, -100.2362) (-24.8397, -100.0364) (-24.6399, -100.0364) knots 0 0 0 1 1 1
  line L1332 (-24.8397, -100.2362) -> (-24.8397, -100.0364) construction
  line L1333 (-24.8397, -100.0364) -> (-24.6399, -100.0364) construction
  spline S373 degree 2 poles (-24.6399, -100.0364) (-24.44, -100.0364) (-24.44, -100.2362) knots 0 0 0 1 1 1
  line L1334 (-24.6399, -100.0364) -> (-24.44, -100.0364) construction
  line L1335 (-24.44, -100.0364) -> (-24.44, -100.2362) construction
  line L1336 (-24.44, -100.2362) -> (-24.44, -102.6276)
  spline S374 degree 2 poles (-24.44, -102.6276) (-24.44, -102.8274) (-24.6399, -102.8274) knots 0 0 0 1 1 1
  line L1337 (-24.44, -102.6276) -> (-24.44, -102.8274) construction
  line L1338 (-24.44, -102.8274) -> (-24.6399, -102.8274) construction
  spline S375 degree 2 poles (-21.8455, -100.2762) (-21.649, -100.486) (-21.649, -100.8324) knots 0 0 0 1 1 1
  line L1339 (-21.8455, -100.2762) -> (-21.649, -100.486) construction
  line L1340 (-21.649, -100.486) -> (-21.649, -100.8324) construction
  line L1341 (-21.649, -100.8324) -> (-21.649, -102.0314)
  spline S376 degree 2 poles (-21.649, -102.0314) (-21.649, -102.3611) (-22.1153, -102.8274) (-22.445, -102.8274) knots 0 0 0 1 2 2 2
  line L1342 (-21.649, -102.0314) -> (-21.649, -102.3611) construction
  line L1343 (-21.649, -102.3611) -> (-22.1153, -102.8274) construction
  line L1344 (-22.1153, -102.8274) -> (-22.445, -102.8274) construction
  line L1345 (-22.445, -102.8274) -> (-22.8447, -102.8274)
  spline S377 degree 2 poles (-22.8447, -102.8274) (-23.1711, -102.8274) (-23.6407, -102.3611) (-23.6407, -102.0314) knots 0 0 0 1 2 2 2
  line L1346 (-22.8447, -102.8274) -> (-23.1711, -102.8274) construction
  line L1347 (-23.1711, -102.8274) -> (-23.6407, -102.3611) construction
  line L1348 (-23.6407, -102.3611) -> (-23.6407, -102.0314) construction
  line L1349 (-23.6407, -102.0314) -> (-23.6407, -99.5568)
  spline S378 degree 2 poles (-23.6407, -99.5568) (-23.6407, -99.2204) (-23.4175, -99.0206) knots 0 0 0 1 1 1
  line L1350 (-23.6407, -99.5568) -> (-23.6407, -99.2204) construction
  line L1351 (-23.6407, -99.2204) -> (-23.4175, -99.0206) construction
  spline S379 degree 2 poles (-23.4175, -99.0206) (-23.2144, -98.8407) (-22.918, -98.8407) knots 0 0 0 1 1 1
  line L1352 (-23.4175, -99.0206) -> (-23.2144, -98.8407) construction
  line L1353 (-23.2144, -98.8407) -> (-22.918, -98.8407) construction
  spline S380 degree 2 poles (-22.918, -98.8407) (-22.6282, -98.8407) (-22.4284, -99.0172) knots 0 0 0 1 1 1
  line L1354 (-22.918, -98.8407) -> (-22.6282, -98.8407) construction
  line L1355 (-22.6282, -98.8407) -> (-22.4284, -99.0172) construction
  spline S381 degree 2 poles (-22.4284, -99.0172) (-22.2052, -99.2171) (-22.2052, -99.5534) knots 0 0 0 1 1 1
  line L1356 (-22.4284, -99.0172) -> (-22.2052, -99.2171) construction
  line L1357 (-22.2052, -99.2171) -> (-22.2052, -99.5534) construction
  spline S382 degree 2 poles (-22.2052, -99.5534) (-22.2052, -99.8898) (-22.445, -100.0497) knots 0 0 0 1 1 1
  line L1358 (-22.2052, -99.5534) -> (-22.2052, -99.8898) construction
  line L1359 (-22.2052, -99.8898) -> (-22.445, -100.0497) construction
  spline S383 degree 2 poles (-22.445, -100.0497) (-22.0587, -100.0497) (-21.8455, -100.2762) knots 0 0 0 1 1 1
  line L1360 (-22.445, -100.0497) -> (-22.0587, -100.0497) construction
  line L1361 (-22.0587, -100.0497) -> (-21.8455, -100.2762) construction
  spline S384 degree 2 poles (-32.4746, -2.8867) (-32.8799, -2.8867) (-33.4722, -2.306) (-33.4722, -1.889) knots 0 0 0 1 2 2 2
  line L1362 (-32.4746, -2.8867) -> (-32.8799, -2.8867) construction
  line L1363 (-32.8799, -2.8867) -> (-33.4722, -2.306) construction
  line L1364 (-33.4722, -2.306) -> (-33.4722, -1.889) construction
  line L1365 (-33.4722, -1.889) -> (-33.4722, 1.104)
  spline S385 degree 2 poles (-33.4722, 1.104) (-33.4722, 1.5209) (-32.8916, 2.1016) (-32.4746, 2.1016) knots 0 0 0 1 2 2 2
  line L1366 (-33.4722, 1.104) -> (-33.4722, 1.5209) construction
  line L1367 (-33.4722, 1.5209) -> (-32.8916, 2.1016) construction
  line L1368 (-32.8916, 2.1016) -> (-32.4746, 2.1016) construction
  line L1369 (-32.4746, 2.1016) -> (-31.2275, 2.1016)
  spline S386 degree 2 poles (-31.2275, 2.1016) (-31.1262, 2.1016) (-30.9781, 1.9496) (-30.9781, 1.8522) knots 0 0 0 1 2 2 2
  line L1370 (-31.2275, 2.1016) -> (-31.1262, 2.1016) construction
  line L1371 (-31.1262, 2.1016) -> (-30.9781, 1.9496) construction
  line L1372 (-30.9781, 1.9496) -> (-30.9781, 1.8522) construction
  spline S387 degree 2 poles (-30.9781, 1.8522) (-30.9781, 1.7665) (-31.1028, 1.6028) (-31.2275, 1.6028) knots 0 0 0 1 2 2 2
  line L1373 (-30.9781, 1.8522) -> (-30.9781, 1.7665) construction
  line L1374 (-30.9781, 1.7665) -> (-31.1028, 1.6028) construction
  line L1375 (-31.1028, 1.6028) -> (-31.2275, 1.6028) construction
  line L1376 (-31.2275, 1.6028) -> (-32.4746, 1.6028)
  spline S388 degree 2 poles (-32.4746, 1.6028) (-32.685, 1.6028) (-32.8292, 1.4586) knots 0 0 0 1 1 1
  line L1377 (-32.4746, 1.6028) -> (-32.685, 1.6028) construction
  line L1378 (-32.685, 1.6028) -> (-32.8292, 1.4586) construction
  spline S389 degree 2 poles (-32.8292, 1.4586) (-32.9033, 1.3884) (-32.9734, 1.2092) (-32.9734, 1.104) knots 0 0 0 1 2 2 2
  line L1379 (-32.8292, 1.4586) -> (-32.9033, 1.3884) construction
  line L1380 (-32.9033, 1.3884) -> (-32.9734, 1.2092) construction
  line L1381 (-32.9734, 1.2092) -> (-32.9734, 1.104) construction
  line L1382 (-32.9734, 1.104) -> (-32.9734, -1.889)
  spline S390 degree 2 poles (-32.9734, -1.889) (-32.9734, -2.0995) (-32.8292, -2.2437) knots 0 0 0 1 1 1
  line L1383 (-32.9734, -1.889) -> (-32.9734, -2.0995) construction
  line L1384 (-32.9734, -2.0995) -> (-32.8292, -2.2437) construction
  spline S391 degree 2 poles (-32.8292, -2.2437) (-32.7552, -2.3099) (-32.6694, -2.3528) knots 0 0 0 1 1 1
  line L1385 (-32.8292, -2.2437) -> (-32.7552, -2.3099) construction
  line L1386 (-32.7552, -2.3099) -> (-32.6694, -2.3528) construction
  spline S392 degree 2 poles (-32.6694, -2.3528) (-32.5642, -2.3879) (-32.4746, -2.3879) knots 0 0 0 1 1 1
  line L1387 (-32.6694, -2.3528) -> (-32.5642, -2.3879) construction
  line L1388 (-32.5642, -2.3879) -> (-32.4746, -2.3879) construction
  line L1389 (-32.4746, -2.3879) -> (-31.2275, -2.3879)
  spline S393 degree 2 poles (-31.2275, -2.3879) (-31.1262, -2.3879) (-30.9781, -2.5398) (-30.9781, -2.6373) knots 0 0 0 1 2 2 2
  line L1390 (-31.2275, -2.3879) -> (-31.1262, -2.3879) construction
  line L1391 (-31.1262, -2.3879) -> (-30.9781, -2.5398) construction
  line L1392 (-30.9781, -2.5398) -> (-30.9781, -2.6373) construction
  spline S394 degree 2 poles (-30.9781, -2.6373) (-30.9781, -2.723) (-31.1028, -2.8867) (-31.2275, -2.8867) knots 0 0 0 1 2 2 2
  line L1393 (-30.9781, -2.6373) -> (-30.9781, -2.723) construction
  line L1394 (-30.9781, -2.723) -> (-31.1028, -2.8867) construction
  line L1395 (-31.1028, -2.8867) -> (-31.2275, -2.8867) construction
  line L1396 (-31.2275, -2.8867) -> (-32.4746, -2.8867)
  spline S395 degree 2 poles (-23.5658, -2.8243) (-23.6359, -2.8867) (-23.745, -2.8867) knots 0 0 0 1 1 1
  line L1397 (-23.5658, -2.8243) -> (-23.6359, -2.8867) construction
  line L1398 (-23.6359, -2.8867) -> (-23.745, -2.8867) construction
  spline S396 degree 2 poles (-23.745, -2.8867) (-23.8464, -2.8867) (-23.9945, -2.762) (-23.9945, -2.6373) knots 0 0 0 1 2 2 2
  line L1399 (-23.745, -2.8867) -> (-23.8464, -2.8867) construction
  line L1400 (-23.8464, -2.8867) -> (-23.9945, -2.762) construction
  line L1401 (-23.9945, -2.762) -> (-23.9945, -2.6373) construction
  spline S397 degree 2 poles (-25.9898, -2.6373) (-25.9898, -2.7542) (-26.0599, -2.8243) knots 0 0 0 1 1 1
  line L1402 (-25.9898, -2.6373) -> (-25.9898, -2.7542) construction
  line L1403 (-25.9898, -2.7542) -> (-26.0599, -2.8243) construction
  spline S398 degree 2 poles (-26.0599, -2.8243) (-26.1301, -2.8867) (-26.2392, -2.8867) knots 0 0 0 1 1 1
  line L1404 (-26.0599, -2.8243) -> (-26.1301, -2.8867) construction
  line L1405 (-26.1301, -2.8867) -> (-26.2392, -2.8867) construction
  spline S399 degree 2 poles (-26.2392, -2.8867) (-26.3405, -2.8867) (-26.4886, -2.762) (-26.4886, -2.6373) knots 0 0 0 1 2 2 2
  line L1406 (-26.2392, -2.8867) -> (-26.3405, -2.8867) construction
  line L1407 (-26.3405, -2.8867) -> (-26.4886, -2.762) construction
  line L1408 (-26.4886, -2.762) -> (-26.4886, -2.6373) construction
  line L1409 (-26.4886, -2.6373) -> (-26.4886, 1.8522)
  spline S400 degree 2 poles (-26.4886, 1.8522) (-26.4886, 2.1016) (-26.2392, 2.1016) knots 0 0 0 1 1 1
  line L1410 (-26.4886, 1.8522) -> (-26.4886, 2.1016) construction
  line L1411 (-26.4886, 2.1016) -> (-26.2392, 2.1016) construction
  line L1412 (-26.2392, 2.1016) -> (-23.745, 2.1016)
  spline S401 degree 2 poles (-23.745, 2.1016) (-23.4956, 2.1016) (-23.4956, 1.8522) knots 0 0 0 1 1 1
  line L1413 (-23.745, 2.1016) -> (-23.4956, 2.1016) construction
  line L1414 (-23.4956, 2.1016) -> (-23.4956, 1.8522) construction
  line L1415 (-23.4956, 1.8522) -> (-23.4956, -2.6373)
  spline S402 degree 2 poles (-23.4956, -2.6373) (-23.4956, -2.7542) (-23.5658, -2.8243) knots 0 0 0 1 1 1
  line L1416 (-23.4956, -2.6373) -> (-23.4956, -2.7542) construction
  line L1417 (-23.4956, -2.7542) -> (-23.5658, -2.8243) construction
  spline S403 degree 2 poles (-2.6579, -39.147) (-3.1442, -39.147) (-3.8551, -38.4502) (-3.8551, -37.9498) knots 0 0 0 1 2 2 2
  line L1418 (-2.6579, -39.147) -> (-3.1442, -39.147) construction
  line L1419 (-3.1442, -39.147) -> (-3.8551, -38.4502) construction
  line L1420 (-3.8551, -38.4502) -> (-3.8551, -37.9498) construction
  line L1421 (-3.8551, -37.9498) -> (-3.8551, -35.8547)
  spline S404 degree 2 poles (-3.8551, -35.8547) (-3.8551, -35.7331) (-3.7662, -35.6302) knots 0 0 0 1 1 1
  line L1422 (-3.8551, -35.8547) -> (-3.8551, -35.7331) construction
  line L1423 (-3.8551, -35.7331) -> (-3.7662, -35.6302) construction
  spline S405 degree 2 poles (-3.7662, -35.6302) (-3.6774, -35.5554) (-3.5558, -35.5554) knots 0 0 0 1 1 1
  line L1424 (-3.7662, -35.6302) -> (-3.6774, -35.5554) construction
  line L1425 (-3.6774, -35.5554) -> (-3.5558, -35.5554) construction
  spline S406 degree 2 poles (-3.5558, -35.5554) (-3.4389, -35.5554) (-3.2565, -35.7051) (-3.2565, -35.8547) knots 0 0 0 1 2 2 2
  line L1426 (-3.5558, -35.5554) -> (-3.4389, -35.5554) construction
  line L1427 (-3.4389, -35.5554) -> (-3.2565, -35.7051) construction
  line L1428 (-3.2565, -35.7051) -> (-3.2565, -35.8547) construction
  line L1429 (-3.2565, -35.8547) -> (-3.2565, -37.9498)
  spline S407 degree 2 poles (-3.2565, -37.9498) (-3.2565, -38.2023) (-3.0834, -38.3754) knots 0 0 0 1 1 1
  line L1430 (-3.2565, -37.9498) -> (-3.2565, -38.2023) construction
  line L1431 (-3.2565, -38.2023) -> (-3.0834, -38.3754) construction
  spline S408 degree 2 poles (-3.0834, -38.3754) (-2.9946, -38.4549) (-2.8917, -38.5063) knots 0 0 0 1 1 1
  line L1432 (-3.0834, -38.3754) -> (-2.9946, -38.4549) construction
  line L1433 (-2.9946, -38.4549) -> (-2.8917, -38.5063) construction
  spline S409 degree 2 poles (-2.8917, -38.5063) (-2.7654, -38.5484) (-2.6579, -38.5484) knots 0 0 0 1 1 1
  line L1434 (-2.8917, -38.5063) -> (-2.7654, -38.5484) construction
  line L1435 (-2.7654, -38.5484) -> (-2.6579, -38.5484) construction
  spline S410 degree 2 poles (-0.8621, -35.8547) (-0.8621, -35.7331) (-0.7732, -35.6302) knots 0 0 0 1 1 1
  line L1436 (-0.8621, -35.8547) -> (-0.8621, -35.7331) construction
  line L1437 (-0.8621, -35.7331) -> (-0.7732, -35.6302) construction
  spline S411 degree 2 poles (-0.7732, -35.6302) (-0.6844, -35.5554) (-0.5628, -35.5554) knots 0 0 0 1 1 1
  line L1438 (-0.7732, -35.6302) -> (-0.6844, -35.5554) construction
  line L1439 (-0.6844, -35.5554) -> (-0.5628, -35.5554) construction
  spline S412 degree 2 poles (-0.5628, -35.5554) (-0.4459, -35.5554) (-0.2635, -35.7051) (-0.2635, -35.8547) knots 0 0 0 1 2 2 2
  line L1440 (-0.5628, -35.5554) -> (-0.4459, -35.5554) construction
  line L1441 (-0.4459, -35.5554) -> (-0.2635, -35.7051) construction
  line L1442 (-0.2635, -35.7051) -> (-0.2635, -35.8547) construction
  line L1443 (-0.2635, -35.8547) -> (-0.2635, -40.3442)
  spline S413 degree 2 poles (-0.2635, -40.3442) (-0.2635, -40.8352) (-0.965, -41.5414) (-1.4607, -41.5414) knots 0 0 0 1 2 2 2
  line L1444 (-0.2635, -40.3442) -> (-0.2635, -40.8352) construction
  line L1445 (-0.2635, -40.8352) -> (-0.965, -41.5414) construction
  line L1446 (-0.965, -41.5414) -> (-1.4607, -41.5414) construction
  line L1447 (-1.4607, -41.5414) -> (-2.9572, -41.5414)
  spline S414 degree 2 poles (-2.9572, -41.5414) (-3.0928, -41.5414) (-3.1816, -41.4572) knots 0 0 0 1 1 1
  line L1448 (-2.9572, -41.5414) -> (-3.0928, -41.5414) construction
  line L1449 (-3.0928, -41.5414) -> (-3.1816, -41.4572) construction
  spline S415 degree 2 poles (-3.1816, -41.4572) (-3.2565, -41.3684) (-3.2565, -41.2421) knots 0 0 0 1 1 1
  line L1450 (-3.1816, -41.4572) -> (-3.2565, -41.3684) construction
  line L1451 (-3.2565, -41.3684) -> (-3.2565, -41.2421) construction
  spline S416 degree 2 poles (-3.2565, -41.2421) (-3.2565, -41.1345) (-3.0975, -40.9428) (-2.9572, -40.9428) knots 0 0 0 1 2 2 2
  line L1452 (-3.2565, -41.2421) -> (-3.2565, -41.1345) construction
  line L1453 (-3.2565, -41.1345) -> (-3.0975, -40.9428) construction
  line L1454 (-3.0975, -40.9428) -> (-2.9572, -40.9428) construction
  line L1455 (-2.9572, -40.9428) -> (-1.4607, -40.9428)
  spline S417 degree 2 poles (-1.4607, -40.9428) (-1.2128, -40.9428) (-0.8621, -40.6108) (-0.8621, -40.3442) knots 0 0 0 1 2 2 2
  line L1456 (-1.4607, -40.9428) -> (-1.2128, -40.9428) construction
  line L1457 (-1.2128, -40.9428) -> (-0.8621, -40.6108) construction
  line L1458 (-0.8621, -40.6108) -> (-0.8621, -40.3442) construction
  spline S418 degree 2 poles (8.2385, -35.6349) (8.332, -35.5554) (8.4442, -35.5554) knots 0 0 0 1 1 1
  line L1459 (8.2385, -35.6349) -> (8.332, -35.5554) construction
  line L1460 (8.332, -35.5554) -> (8.4442, -35.5554) construction
  spline S419 degree 2 poles (8.4442, -35.5554) (8.5565, -35.5554) (8.7482, -35.7378) (8.7482, -35.8641) knots 0 0 0 1 2 2 2
  line L1461 (8.4442, -35.5554) -> (8.5565, -35.5554) construction
  line L1462 (8.5565, -35.5554) -> (8.7482, -35.7378) construction
  line L1463 (8.7482, -35.7378) -> (8.7482, -35.8641) construction
  spline S420 degree 2 poles (8.7482, -35.8641) (8.7482, -35.9389) (8.6594, -36.0652) knots 0 0 0 1 1 1
  line L1464 (8.7482, -35.8641) -> (8.7482, -35.9389) construction
  line L1465 (8.7482, -35.9389) -> (8.6594, -36.0652) construction
  spline S421 degree 2 poles (8.7576, -41.2514) (8.7576, -41.3684) (8.6594, -41.4525) knots 0 0 0 1 1 1
  line L1466 (8.7576, -41.2514) -> (8.7576, -41.3684) construction
  line L1467 (8.7576, -41.3684) -> (8.6594, -41.4525) construction
  spline S422 degree 2 poles (8.6594, -41.4525) (8.5705, -41.5414) (8.4396, -41.5414) knots 0 0 0 1 1 1
  line L1468 (8.6594, -41.4525) -> (8.5705, -41.5414) construction
  line L1469 (8.5705, -41.5414) -> (8.4396, -41.5414) construction
  spline S423 degree 2 poles (8.4396, -41.5414) (8.2946, -41.5414) (8.187, -41.3824) knots 0 0 0 1 1 1
  line L1470 (8.4396, -41.5414) -> (8.2946, -41.5414) construction
  line L1471 (8.2946, -41.5414) -> (8.187, -41.3824) construction
  spline S424 degree 2 poles (5.7225, -41.2421) (5.7225, -41.3824) (5.6383, -41.4666) knots 0 0 0 1 1 1
  line L1472 (5.7225, -41.2421) -> (5.7225, -41.3824) construction
  line L1473 (5.7225, -41.3824) -> (5.6383, -41.4666) construction
  spline S425 degree 2 poles (5.6383, -41.4666) (5.5541, -41.5414) (5.4232, -41.5414) knots 0 0 0 1 1 1
  line L1474 (5.6383, -41.4666) -> (5.5541, -41.5414) construction
  line L1475 (5.5541, -41.5414) -> (5.4232, -41.5414) construction
  spline S426 degree 2 poles (5.4232, -41.5414) (5.3016, -41.5414) (5.1239, -41.3917) (5.1239, -41.2421) knots 0 0 0 1 2 2 2
  line L1476 (5.4232, -41.5414) -> (5.3016, -41.5414) construction
  line L1477 (5.3016, -41.5414) -> (5.1239, -41.3917) construction
  line L1478 (5.1239, -41.3917) -> (5.1239, -41.2421) construction
  line L1479 (5.1239, -41.2421) -> (5.1239, -35.8454)
  spline S427 degree 2 poles (5.1239, -35.8454) (5.1239, -35.7331) (5.3063, -35.5554) (5.4232, -35.5554) knots 0 0 0 1 2 2 2
  line L1480 (5.1239, -35.8454) -> (5.1239, -35.7331) construction
  line L1481 (5.1239, -35.7331) -> (5.3063, -35.5554) construction
  line L1482 (5.3063, -35.5554) -> (5.4232, -35.5554) construction
  spline S428 degree 2 poles (5.4232, -35.5554) (5.5401, -35.5554) (5.6336, -35.6256) knots 0 0 0 1 1 1
  line L1483 (5.4232, -35.5554) -> (5.5401, -35.5554) construction
  line L1484 (5.5401, -35.5554) -> (5.6336, -35.6256) construction
  spline S429 degree 2 poles (5.6336, -35.6256) (5.7225, -35.7004) (5.7225, -35.8454) knots 0 0 0 1 1 1
  line L1485 (5.6336, -35.6256) -> (5.7225, -35.7004) construction
  line L1486 (5.7225, -35.7004) -> (5.7225, -35.8454) construction
  spline S430 degree 2 poles (25.5405, 2.027) (25.4509, 2.1283) (25.4509, 2.2374) knots 0 0 0 1 1 1
  line L1487 (25.5405, 2.027) -> (25.4509, 2.1283) construction
  line L1488 (25.4509, 2.1283) -> (25.4509, 2.2374) construction
  spline S431 degree 2 poles (25.4509, 2.2374) (25.4509, 2.3153) (25.5795, 2.4595) (25.7159, 2.4595) knots 0 0 0 1 2 2 2
  line L1489 (25.4509, 2.2374) -> (25.4509, 2.3153) construction
  line L1490 (25.4509, 2.3153) -> (25.5795, 2.4595) construction
  line L1491 (25.5795, 2.4595) -> (25.7159, 2.4595) construction
  line L1492 (25.7159, 2.4595) -> (27.7112, 2.4595)
  spline S432 degree 2 poles (27.7112, 2.4595) (27.8164, 2.4595) (27.9606, 2.3076) (27.9606, 2.2101) knots 0 0 0 1 2 2 2
  line L1493 (27.7112, 2.4595) -> (27.8164, 2.4595) construction
  line L1494 (27.8164, 2.4595) -> (27.9606, 2.3076) construction
  line L1495 (27.9606, 2.3076) -> (27.9606, 2.2101) construction
  spline S433 degree 2 poles (27.9606, 2.2101) (27.9606, 2.1244) (27.8359, 1.9607) (27.7112, 1.9607) knots 0 0 0 1 2 2 2
  line L1496 (27.9606, 2.2101) -> (27.9606, 2.1244) construction
  line L1497 (27.9606, 2.1244) -> (27.8359, 1.9607) construction
  line L1498 (27.8359, 1.9607) -> (27.7112, 1.9607) construction
  spline S434 degree 2 poles (27.7229, 0.6162) (27.9606, 0.3356) (27.9606, -0.0346) knots 0 0 0 1 1 1
  line L1499 (27.7229, 0.6162) -> (27.9606, 0.3356) construction
  line L1500 (27.9606, 0.3356) -> (27.9606, -0.0346) construction
  line L1501 (27.9606, -0.0346) -> (27.9606, -1.5311)
  spline S435 degree 2 poles (27.9606, -1.5311) (27.9606, -1.9403) (27.376, -2.5288) (26.9629, -2.5288) knots 0 0 0 1 2 2 2
  line L1502 (27.9606, -1.5311) -> (27.9606, -1.9403) construction
  line L1503 (27.9606, -1.9403) -> (27.376, -2.5288) construction
  line L1504 (27.376, -2.5288) -> (26.9629, -2.5288) construction
  line L1505 (26.9629, -2.5288) -> (26.4641, -2.5288)
  spline S436 degree 2 poles (26.4641, -2.5288) (26.0627, -2.5288) (25.4664, -1.952) (25.4664, -1.5311) knots 0 0 0 1 2 2 2
  line L1506 (26.4641, -2.5288) -> (26.0627, -2.5288) construction
  line L1507 (26.0627, -2.5288) -> (25.4664, -1.952) construction
  line L1508 (25.4664, -1.952) -> (25.4664, -1.5311) construction
  line L1509 (25.4664, -1.5311) -> (25.4664, -0.0346)
  spline S437 degree 2 poles (25.4664, -0.0346) (25.4664, 0.3785) (26.051, 0.963) (26.4641, 0.963) knots 0 0 0 1 2 2 2
  line L1510 (25.4664, -0.0346) -> (25.4664, 0.3785) construction
  line L1511 (25.4664, 0.3785) -> (26.051, 0.963) construction
  line L1512 (26.051, 0.963) -> (26.4641, 0.963) construction
  spline S438 degree 2 poles (29.4571, -3.7758) (29.4571, -3.8811) (29.3051, -4.0253) (29.2077, -4.0253) knots 0 0 0 1 2 2 2
  line L1513 (29.4571, -3.7758) -> (29.4571, -3.8811) construction
  line L1514 (29.4571, -3.8811) -> (29.3051, -4.0253) construction
  line L1515 (29.3051, -4.0253) -> (29.2077, -4.0253) construction
  spline S439 degree 2 poles (29.2077, -4.0253) (29.1219, -4.0253) (28.9583, -3.9006) (28.9583, -3.7758) knots 0 0 0 1 2 2 2
  line L1516 (29.2077, -4.0253) -> (29.1219, -4.0253) construction
  line L1517 (29.1219, -4.0253) -> (28.9583, -3.9006) construction
  line L1518 (28.9583, -3.9006) -> (28.9583, -3.7758) construction
  line L1519 (28.9583, -3.7758) -> (28.9583, 0.7136)
  spline S440 degree 2 poles (28.9583, 0.7136) (28.9583, 0.963) (29.2077, 0.963) knots 0 0 0 1 1 1
  line L1520 (28.9583, 0.7136) -> (28.9583, 0.963) construction
  line L1521 (28.9583, 0.963) -> (29.2077, 0.963) construction
  line L1522 (29.2077, 0.963) -> (30.4548, 0.963)
  spline S441 degree 2 poles (30.4548, 0.963) (30.8601, 0.963) (31.4524, 0.3824) (31.4524, -0.0346) knots 0 0 0 1 2 2 2
  line L1523 (30.4548, 0.963) -> (30.8601, 0.963) construction
  line L1524 (30.8601, 0.963) -> (31.4524, 0.3824) construction
  line L1525 (31.4524, 0.3824) -> (31.4524, -0.0346) construction
  line L1526 (31.4524, -0.0346) -> (31.4524, -1.5311)
  spline S442 degree 2 poles (31.4524, -1.5311) (31.4524, -1.9403) (30.8678, -2.5288) (30.4548, -2.5288) knots 0 0 0 1 2 2 2
  line L1527 (31.4524, -1.5311) -> (31.4524, -1.9403) construction
  line L1528 (31.4524, -1.9403) -> (30.8678, -2.5288) construction
  line L1529 (30.8678, -2.5288) -> (30.4548, -2.5288) construction
  line L1530 (33.8452, -2.5288) -> (33.5491, -2.5288)
  spline S443 degree 2 poles (33.5491, -2.5288) (33.1009, -2.5288) (32.4501, -1.8935) (32.4501, -1.4298) knots 0 0 0 1 2 2 2
  line L1531 (33.5491, -2.5288) -> (33.1009, -2.5288) construction
  line L1532 (33.1009, -2.5288) -> (32.4501, -1.8935) construction